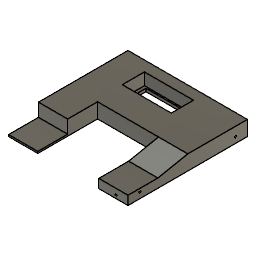
Front - Structure (Autodesk Fusion 360 design; units mm, degrees)
part number: 2026-03-10-09-19-59-139
Autodesk Fusion 360 part; units mm, degrees
sketch "Esquisse2" plane through (0, 0, 0) normal (0, 0, 1) x (1, 0, 0)
  line L0 (200, 0) -> (200, 200)
  line L1 (200, 200) -> (0, 200)
  line L2 (0, 200) -> (0, 0)
  line L3 (151, 0) -> (151, 100)
  line L4 (151, 100) -> (49, 100)
  line L5 (49, 100) -> (49, 0)
  line L6 (50, 180) -> (120, 180)
  line L7 (120, 180) -> (120, 155)
  line L8 (120, 155) -> (50, 155)
  line L9 (50, 155) -> (50, 180)
  line L10 (0, 0) -> (49, 0)
  line L11 (151, 0) -> (200, 0)
  line L12 (45, 152.5) -> (125, 152.5)
  line L13 (125, 152.5) -> (125, 182.5)
  line L14 (125, 182.5) -> (45, 182.5)
  line L15 (45, 182.5) -> (45, 152.5)
  point P0 (45, 180)
  point P1 (45, 152.5)
  dimension "d8" = 200
  dimension "d10" = 100
  dimension "d12" = 70
  dimension "d13" = 25
  dimension "d27" = 5
  dimension "d30" = 80
  dimension "d31" = 30
  dimension "d37" = 49
  dimension "d38" = 49
  dimension "d39" = 102
  constraint vertical L0
  constraint horizontal L1
  constraint vertical L2
  constraint coincident L2.end L10.start
  constraint vertical L3
  constraint horizontal L4
  constraint vertical L5
  constraint horizontal L6
  constraint vertical L7
  constraint horizontal L8
  constraint vertical L9
  constraint perpendicular L5 L10
  constraint perpendicular L0 L11
  constraint horizontal L12
  constraint vertical L13
  constraint horizontal L14
  constraint vertical L15
  constraint coincident P1 L12.start
  measures "d8" distance of L2.end L1.end
  measures "d10" distance of L5.end L4.end
  measures "d12" distance of L6.start L6.end
  measures "d13" distance of L6.start L8.end
  measures "d27" distance of L6.start P0
  measures "d30" distance of P1 L12.end
  measures "d31" distance of P1 L14.end
  measures "d37" distance of L2 L5
  measures "d38" distance of L0 L3
  measures "d39" distance of L5.end L3.start
extrude "Extrusion2" add sketch "Esquisse2" along normal blind 25 contours L0 L1 L2 L3 L4 L5 L10 L11 | L12 L13 L14 L15
ref_plane "Plan de construction1" through (85, 167.5, 30) normal (0, 0, 1) x (1, 0, 0)
sketch "Esquisse7" plane through (0, 0, 30) normal (0, 0, 1) x (1, 0, 0)
  line L0 (45, 182.5) -> (127, 182.5)
  line L1 (127, 182.5) -> (127, 145.5)
  line L2 (127, 145.5) -> (45, 145.5)
  line L3 (45, 145.5) -> (45, 182.5)
  dimension "d33" = 82
  dimension "d34" = 37
  constraint horizontal L0
  constraint vertical L1
  constraint horizontal L2
  constraint vertical L3
  measures "d33" distance of L0.start L0.end
  measures "d34" distance of L0.start L2.end
extrude "Extrusion5" cut sketch "Esquisse7" against normal blind 25
sketch "Esquisse8" plane through (200, 0, 0) normal (1, 0, 0) x (0, 1, 0)
  line L0 (0, 0) -> (200, 0)
  line L1 (200, 0) -> (200, 25)
  line L2 (200, 25) -> (0, 25)
  line L3 (0, 25) -> (0, 0)
  circle A0 centre (180, 10) radius 2
  circle A1 centre (20, 10) radius 2
  point P0 (180, 10)
  point P1 (20, 10)
  dimension "d40" = 20
  dimension "d41" = 20
  dimension "d42" = 4
  dimension "d43" = 4
  constraint coincident P0 A0.centre
  constraint coincident P1 A1.centre
  measures "d40" distance of L1 P0
  measures "d41" distance of L3 P1
  measures "d42" diameter of A0
  measures "d43" diameter of A1
extrude "Extrusion6" cut sketch "Esquisse8" against normal blind 20 contours A0 | A1
thread "Filetage1" "ISO Metric profile 4.0 M4x0.7 M4x0.7 6H" major diameter 4.1095 minor diameter 3.332 pitch 0.7 angle 60 resizes the face on face at (193.3333, 179.0876, 8.2203) on face at (186.6667, 21.9975, 9.9003)
sketch "Esquisse9" plane through (0, 0, 0) normal (-1, 0, 0) x (0, -1, 0)
  line L0 (-200, 0) -> (0, 0)
  line L1 (0, 0) -> (0, 25)
  line L2 (0, 25) -> (-200, 25)
  line L3 (-200, 25) -> (-200, 0)
  circle A0 centre (-180, 10) radius 2
  point P0 (-180, 10)
  point P1 (-20, 10)
  dimension "d48" = 20
  dimension "d49" = 20
  dimension "d50" = 4
  constraint coincident P0 A0.centre
  measures "d48" distance of L1 P1
  measures "d49" distance of L3 P0
  measures "d50" diameter of A0
extrude "Extrusion7" cut sketch "Esquisse9" against normal blind 15 contours A0
sketch "Esquisse10" plane through (0, 0, 0) normal (0, -1, 0) x (1, 0, 0)
  line L0 (0, 0) -> (49, 0)
  line L1 (49, 0) -> (49, 25)
  line L2 (49, 25) -> (0, 25)
  line L3 (0, 25) -> (0, 0)
  line L4 (200, 0) -> (200, 25)
  line L5 (151, 25) -> (200, 25)
  circle A0 centre (180, 5) radius 2
  point P0 (20, 5)
  point P1 (180, 5)
  dimension "d57" = 20
  dimension "d58" = 20
  dimension "d59" = 20
  dimension "d60" = 20
  dimension "d61" = 4
  constraint coincident P1 A0.centre
  measures "d57" distance of L3 P0
  measures "d58" distance of L2 P0
  measures "d59" distance of P1 L4
  measures "d60" distance of P1 L5
  measures "d61" diameter of A0
extrude "Extrusion8" cut sketch "Esquisse10" against normal blind 15 contours A0
sketch "Esquisse12" plane through (200, 0, 0) normal (1, 0, 0) x (0, 1, 0)
  circle A0 centre (180, 10) radius 1.666
  circle A1 centre (20, 10) radius 1.666
  line L0 (0, 0) -> (200, 0)
  line L1 (200, 0) -> (200, 25)
  line L2 (200, 25) -> (0, 25)
  line L3 (0, 25) -> (0, 0)
  line L4 (0, 25) -> (50, 25)
  line L5 (50, 25) -> (50, 15)
  line L6 (50, 15) -> (0, 15)
  line L7 (0, 15) -> (0, 25)
  dimension "d70" = 50
  dimension "d71" = 10
  constraint horizontal L4
  constraint vertical L5
  constraint horizontal L6
  constraint vertical L7
  constraint coincident L2.end L3.start
  measures "d70" distance of L2.end L4.end
  measures "d71" distance of L2.end L6.end
extrude "Extrusion10" cut sketch "Esquisse12" against normal blind 50 contours L2 L3 L4 L5 L6 L7
chamfer "Chanfrein2" distance 50 distance2 10 1 edges at (175.5, 50, 25) measured on face at (16.3333, 100, 25)
sketch "Esquisse13" plane through (0, 0, 0) normal (-1, 0, 0) x (0, -1, 0)
  circle A0 centre (-180, 10) radius 2
  line L0 (-200, 0) -> (0, 0)
  line L1 (0, 0) -> (0, 25)
  line L2 (0, 25) -> (-200, 25)
  line L3 (-200, 25) -> (-200, 0)
  line L4 (0, 25) -> (-50, 25)
  line L5 (-50, 25) -> (-50, 3)
  line L6 (-50, 3) -> (0, 3)
  line L7 (0, 3) -> (0, 25)
  dimension "d76" = 50
  dimension "d77" = 22
  constraint horizontal L4
  constraint vertical L5
  constraint horizontal L6
  constraint vertical L7
  constraint coincident L1.end L2.start
  measures "d76" distance of L1.end L4.end
  measures "d77" distance of L1.end L6.end
extrude "Extrusion11" cut sketch "Esquisse13" against normal blind 50 contours L1 L2 L4 L5 L6 L7
thread "Filetage4" "ISO Metric profile 4.0 M4x0.7 M4x0.7 6H" major diameter 4.1095 minor diameter 3.332 pitch 0.7 angle 60 resizes the face on face at (179.0876, 10, 3.2203) on face at (10, 178.6766, 11.4996)
move_face "DécalerLesFaces1" offset -0.05 4 faces at (10, 178.672, 11.0059) (179.4694, 5, 3.4208) (186.6667, 21.6639, 9.917) (186.6667, 181.328, 11.0059)
